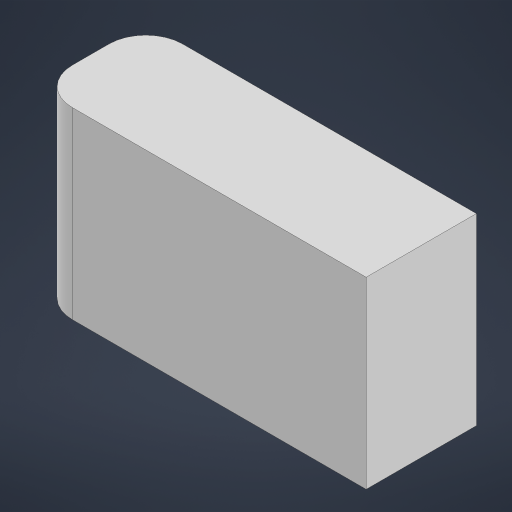
# Autodesk Inventor part: 2s lipo
Saved by Autodesk Inventor 2024 (Build 280153000, 153)
## iProperties
Created: 2024-02-09
Part Number: 2s lipo
Material: Všeobecné
Document SubType Name: Modeling
Designer: Simak
Density: 1 g/cm^3
Appearance: Výchozí
Author: Simak
Autodesk Inventor part; units mm, degrees
ref_plane "YZ Plane" through (0, 0, 0) normal (1, 0, 0) x (0, 1, 0)
ref_plane "XZ Plane" through (0, 0, 0) normal (0, 1, 0) x (-1, 0, 0)
ref_plane "XY Plane" through (0, 0, 0) normal (0, 0, 1) x (1, 0, 0)
sketch "Náčrt1" plane through (0, 0, 0) normal (0, 1, 0) x (-1, 0, 0)
  line L0 (40, 0) -> (0, 0)
  line L1 (0, 0) -> (0, -15)
  line L2 (0, -15) -> (40, -15)
  arc A0 (40, -15) -> (45, -10) centre (40, -10) ccw
  line L3 (45, -10) -> (45, -5)
  arc A1 (45, -5) -> (40, 0) centre (40, -5) ccw
  dimension "d0" = 15
  dimension "d1" = 45
  dimension "d2" = 5
  constraints: 8 end point, 4 point on circle, 4 tangent, 3 perpendicular, 2 centre point, 1 coincident, 1 equal radius, 1 horizontal
  measures "d0" distance of L0.end L1.end
  measures "d1" distance between parallel lines of L1 L3
  measures "d2" distance of L3.start L3.end
extrude "Vysunutí1" add sketch "Náčrt1" along normal blind 25
